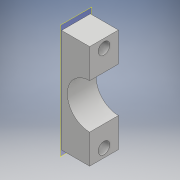
# Autodesk Inventor part: mounpt2
Saved by Autodesk Inventor 2018 (Build 220112000, 112)
## iProperties
Created: 2017-06-25
Part Number: mounpt2
Material: Generic
Document SubType Name: Modeling
Designer: Zadeka
Density: 1 g/cm^3
Appearance: Default
Author: Zadeka
Autodesk Inventor part; units mm, degrees
ref_plane "YZ Plane" through (0, 0, 0) normal (1, 0, 0) x (0, 1, 0)
ref_plane "XZ Plane" through (0, 0, 0) normal (0, 1, 0) x (-1, 0, 0)
ref_plane "XY Plane" through (0, 0, 0) normal (0, 0, 1) x (1, 0, 0)
sketch "Sketch3" plane through (0, 0, 0) normal (0, 1, 0) x (-1, 0, 0)
  arc A0 (0, -15.5) -> (0, 15.5) centre (0, 0) ccw
  line L0 (0, 15.5) -> (0, 36)
  line L1 (0, -15.5) -> (0, -36)
  line L2 (0, 36) -> (19.5, 36)
  line L3 (19.5, 36) -> (19.5, -36)
  line L4 (19.5, -36) -> (0, -36)
  dimension "d17" = 31
  dimension "d19" = 20.5
  dimension "d20" = 20.5
  constraints: 10 end point, 2 perpendicular, 2 point on circle, 2 vertical, 1 centre point, 1 coincident
  measures "d17" diameter of A0
  measures "d19" distance of L0.start L0.end
  measures "d20" distance of L1.start L1.end
extrude "Extrusion3" add sketch "Sketch3" along normal blind 20
ref_plane "Work Plane2" through (-19.5, 0, -36) normal (-1, 0, 0) x (0, 0, 1)
sketch "Sketch4" plane through (-19.5, 0, -36) normal (-1, 0, 0) x (0, 0, 1)
  line L0 (0, 0) -> (0, 20) projected
  line L1 (0, 10) -> (6, 10)
  line L2 (72, 0) -> (72, 20) projected
  line L3 (72, 10) -> (66, 10)
  circle A0 centre (6, 10) radius 4.05
  circle A1 centre (66, 10) radius 4.05
  point P0 (36, 0)
  dimension "d25" = 6
  dimension "d26" = 6
  dimension "d27" = 8.1
  dimension "d28" = 8.1
  constraints: 4 end point, 2 centre point, 2 coincident, 2 horizontal, 2 midpoint
  measures "d25" distance of L1.start L1.end
  measures "d26" distance of L3.start L3.end
  measures "d27" diameter of A0
  measures "d28" diameter of A1
extrude "Extrusion4" cut sketch "Sketch4" against normal blind 20
body "Solid2"
